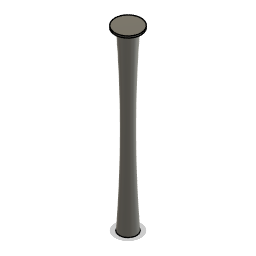
Old_gps mount v2 (Autodesk Fusion 360 design; units mm, degrees)
Autodesk Fusion 360 part; units mm, degrees
sketch "Sketch1" plane through (0, 0, 0) normal (0, 1, 0) x (1, 0, 0)
  circle A0 centre (0, 0) radius 15
  line L0 (5, -10) -> (-5, 10) construction
  line L1 (-5, -10) -> (5, 10) construction
  circle A1 centre (-5, -10) radius 1.5
  circle A2 centre (5, -10) radius 1.5
  circle A3 centre (-5, 10) radius 1.5
  circle A4 centre (5, 10) radius 1.5
  dimension "d10" = 30
  dimension "d29" = 10
  dimension "d30" = 20
  dimension "d31" = 3
  dimension "d32" = 3
  dimension "d33" = 3
  dimension "d34" = 3
  constraint coincident A0.centre origin
  constraint coincident L0 A0.centre
  constraint coincident L1 A0.centre
  constraint coincident L1.start A1.centre
  constraint coincident L0.start A2.centre
  constraint coincident L0.end A3.centre
  constraint coincident L1.end A4.centre
  measures "d10" diameter of A0
  measures "d29" distance of L0.end L1.end
  measures "d30" distance of L1.start L0.end
  measures "d31" diameter of A1
  measures "d32" diameter of A2
  measures "d33" diameter of A3
  measures "d34" diameter of A4
ref_plane "WorkPlane1" through (0, 304.8, 0) normal (0, 1, 0) x (1, 0, 0)
sketch "Sketch2" plane through (0, 304.8, 0) normal (0, 1, 0) x (1, 0, 0)
  circle A0 centre (0, 0) radius 15
  dimension "d16" = 30
  constraint coincident A0.centre origin
  measures "d16" diameter of A0
ref_plane "WorkPlane2" through (0, 152.4, 0) normal (0, 1, 0) x (1, 0, 0)
sketch "Sketch3" plane through (0, 152.4, 0) normal (0, 1, 0) x (1, 0, 0)
  circle A0 centre (0, 0) radius 10
  dimension "d18" = 20
  constraint coincident A0.centre origin
  measures "d18" diameter of A0
loft "Loft1" add profiles "Sketch1", "Sketch3", "Sketch2" section 1 contours A0 | A1 | A2 | A3 | A4 section 2 section 3
sketch "Sketch4" plane through (0, 304.8, 0) normal (0, 1, 0) x (-1, 0, 0)
  circle A0 centre (0, 0) radius 15
  circle A1 centre (0, 0) radius 22.5
  dimension "d21" = 45
  constraint concentric A0 A1
  measures "d21" diameter of A1
extrude "Extrude2" add sketch "Sketch4" along normal blind 3 contours A0 | A1
extrude "Extrude3" cut sketch "Sketch1" along normal blind 10 contours A1 | A2 | A3 | A4
